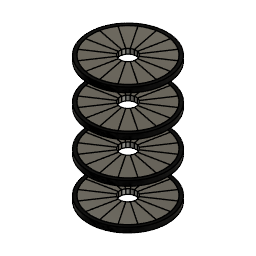
12_seal_stack_assy_set (Autodesk Fusion 360 design; units mm, degrees)
part number: 2026-05-30-09-04-55-823
Autodesk Fusion 360 part; units mm, degrees
ref_plane "WorkPlane1" through (0, 0, 50.165) normal (0, 0, 1) x (1, 0, 0)
sketch "Sketch1" plane through (0, 0, 50.165) normal (0, 0, 1) x (1, 0, 0)
  arc A0 (22.2962, -4.435) -> (22.2962, 4.435) centre (0, 0) ccw
  line L0 (22.2962, 4.435) -> (99.9218, 19.8757)
  arc A1 (99.9218, -19.8757) -> (99.9218, 19.8757) centre (0, 0) ccw
  line L1 (99.9218, -19.8757) -> (22.2962, -4.435)
extrude "Extrude1" add sketch "Sketch1" along normal blind 13.97 makes body 1
ref_plane "WorkPlane2" through (0, 0, 50.165) normal (0, 0, 1) x (1, 0, 0)
sketch "Sketch2" plane through (0, 0, 50.165) normal (0, 0, 1) x (1, 0, 0)
  arc A0 (22.2962, 4.435) -> (18.9018, 12.6298) centre (0, 0) ccw
  line L0 (18.9018, 12.6298) -> (84.7096, 56.6012)
  arc A1 (99.9218, 19.8757) -> (84.7096, 56.6012) centre (0, 0) ccw
  line L1 (99.9218, 19.8757) -> (22.2962, 4.435)
extrude "Extrude2" add sketch "Sketch2" along normal blind 13.97 separate body makes body 2
ref_plane "WorkPlane3" through (0, 0, 50.165) normal (0, 0, 1) x (1, 0, 0)
sketch "Sketch3" plane through (0, 0, 50.165) normal (0, 0, 1) x (1, 0, 0)
  arc A0 (18.9018, 12.6298) -> (12.6298, 18.9018) centre (0, 0) ccw
  line L0 (12.6298, 18.9018) -> (56.6012, 84.7096)
  arc A1 (84.7096, 56.6012) -> (56.6012, 84.7096) centre (0, 0) ccw
  line L1 (84.7096, 56.6012) -> (18.9018, 12.6298)
extrude "Extrude3" add sketch "Sketch3" along normal blind 13.97 separate body makes body 3
ref_plane "WorkPlane4" through (0, 0, 50.165) normal (0, 0, 1) x (1, 0, 0)
sketch "Sketch4" plane through (0, 0, 50.165) normal (0, 0, 1) x (1, 0, 0)
  arc A0 (12.6298, 18.9018) -> (4.435, 22.2962) centre (0, 0) ccw
  line L0 (4.435, 22.2962) -> (19.8757, 99.9218)
  arc A1 (56.6012, 84.7096) -> (19.8757, 99.9218) centre (0, 0) ccw
  line L1 (56.6012, 84.7096) -> (12.6298, 18.9018)
extrude "Extrude4" add sketch "Sketch4" along normal blind 13.97 separate body makes body 4
ref_plane "WorkPlane5" through (0, 0, 50.165) normal (0, 0, 1) x (1, 0, 0)
sketch "Sketch5" plane through (0, 0, 50.165) normal (0, 0, 1) x (1, 0, 0)
  arc A0 (4.435, 22.2962) -> (-4.435, 22.2962) centre (0, 0) ccw
  line L0 (-4.435, 22.2962) -> (-19.8757, 99.9218)
  arc A1 (19.8757, 99.9218) -> (-19.8757, 99.9218) centre (0, 0) ccw
  line L1 (19.8757, 99.9218) -> (4.435, 22.2962)
extrude "Extrude5" add sketch "Sketch5" along normal blind 13.97 separate body makes body 5
ref_plane "WorkPlane6" through (0, 0, 50.165) normal (0, 0, 1) x (1, 0, 0)
sketch "Sketch6" plane through (0, 0, 50.165) normal (0, 0, 1) x (1, 0, 0)
  arc A0 (-4.435, 22.2962) -> (-12.6298, 18.9018) centre (0, 0) ccw
  line L0 (-12.6298, 18.9018) -> (-56.6012, 84.7096)
  arc A1 (-19.8757, 99.9218) -> (-56.6012, 84.7096) centre (0, 0) ccw
  line L1 (-19.8757, 99.9218) -> (-4.435, 22.2962)
extrude "Extrude6" add sketch "Sketch6" along normal blind 13.97 separate body makes body 6
ref_plane "WorkPlane7" through (0, 0, 50.165) normal (0, 0, 1) x (1, 0, 0)
sketch "Sketch7" plane through (0, 0, 50.165) normal (0, 0, 1) x (1, 0, 0)
  arc A0 (-12.6298, 18.9018) -> (-18.9018, 12.6298) centre (0, 0) ccw
  line L0 (-18.9018, 12.6298) -> (-84.7096, 56.6012)
  arc A1 (-56.6012, 84.7096) -> (-84.7096, 56.6012) centre (0, 0) ccw
  line L1 (-56.6012, 84.7096) -> (-12.6298, 18.9018)
extrude "Extrude7" add sketch "Sketch7" along normal blind 13.97 separate body makes body 7
ref_plane "WorkPlane8" through (0, 0, 50.165) normal (0, 0, 1) x (1, 0, 0)
sketch "Sketch8" plane through (0, 0, 50.165) normal (0, 0, 1) x (1, 0, 0)
  arc A0 (-18.9018, 12.6298) -> (-22.2962, 4.435) centre (0, 0) ccw
  line L0 (-22.2962, 4.435) -> (-99.9218, 19.8757)
  arc A1 (-84.7096, 56.6012) -> (-99.9218, 19.8757) centre (0, 0) ccw
  line L1 (-84.7096, 56.6012) -> (-18.9018, 12.6298)
extrude "Extrude8" add sketch "Sketch8" along normal blind 13.97 separate body makes body 8
ref_plane "WorkPlane9" through (0, 0, 50.165) normal (0, 0, 1) x (1, 0, 0)
sketch "Sketch9" plane through (0, 0, 50.165) normal (0, 0, 1) x (1, 0, 0)
  arc A0 (-22.2962, 4.435) -> (-22.2962, -4.435) centre (0, 0) ccw
  line L0 (-22.2962, -4.435) -> (-99.9218, -19.8757)
  arc A1 (-99.9218, 19.8757) -> (-99.9218, -19.8757) centre (0, 0) ccw
  line L1 (-99.9218, 19.8757) -> (-22.2962, 4.435)
extrude "Extrude9" add sketch "Sketch9" along normal blind 13.97 separate body makes body 9
ref_plane "WorkPlane10" through (0, 0, 50.165) normal (0, 0, 1) x (1, 0, 0)
sketch "Sketch10" plane through (0, 0, 50.165) normal (0, 0, 1) x (1, 0, 0)
  arc A0 (-22.2962, -4.435) -> (-18.9018, -12.6298) centre (0, 0) ccw
  line L0 (-18.9018, -12.6298) -> (-84.7096, -56.6012)
  arc A1 (-99.9218, -19.8757) -> (-84.7096, -56.6012) centre (0, 0) ccw
  line L1 (-99.9218, -19.8757) -> (-22.2962, -4.435)
extrude "Extrude10" add sketch "Sketch10" along normal blind 13.97 separate body makes body 10
ref_plane "WorkPlane11" through (0, 0, 50.165) normal (0, 0, 1) x (1, 0, 0)
sketch "Sketch11" plane through (0, 0, 50.165) normal (0, 0, 1) x (1, 0, 0)
  arc A0 (-18.9018, -12.6298) -> (-12.6298, -18.9018) centre (0, 0) ccw
  line L0 (-12.6298, -18.9018) -> (-56.6012, -84.7096)
  arc A1 (-84.7096, -56.6012) -> (-56.6012, -84.7096) centre (0, 0) ccw
  line L1 (-84.7096, -56.6012) -> (-18.9018, -12.6298)
extrude "Extrude11" add sketch "Sketch11" along normal blind 13.97 separate body makes body 11
ref_plane "WorkPlane12" through (0, 0, 50.165) normal (0, 0, 1) x (1, 0, 0)
sketch "Sketch12" plane through (0, 0, 50.165) normal (0, 0, 1) x (1, 0, 0)
  arc A0 (-12.6298, -18.9018) -> (-4.435, -22.2962) centre (0, 0) ccw
  line L0 (-4.435, -22.2962) -> (-19.8757, -99.9218)
  arc A1 (-56.6012, -84.7096) -> (-19.8757, -99.9218) centre (0, 0) ccw
  line L1 (-56.6012, -84.7096) -> (-12.6298, -18.9018)
extrude "Extrude12" add sketch "Sketch12" along normal blind 13.97 separate body makes body 12
ref_plane "WorkPlane13" through (0, 0, 50.165) normal (0, 0, 1) x (1, 0, 0)
sketch "Sketch13" plane through (0, 0, 50.165) normal (0, 0, 1) x (1, 0, 0)
  arc A0 (-4.435, -22.2962) -> (4.435, -22.2962) centre (0, 0) ccw
  line L0 (4.435, -22.2962) -> (19.8757, -99.9218)
  arc A1 (-19.8757, -99.9218) -> (19.8757, -99.9218) centre (0, 0) ccw
  line L1 (-19.8757, -99.9218) -> (-4.435, -22.2962)
extrude "Extrude13" add sketch "Sketch13" along normal blind 13.97 separate body makes body 13
ref_plane "WorkPlane14" through (0, 0, 50.165) normal (0, 0, 1) x (1, 0, 0)
sketch "Sketch14" plane through (0, 0, 50.165) normal (0, 0, 1) x (1, 0, 0)
  arc A0 (4.435, -22.2962) -> (12.6298, -18.9018) centre (0, 0) ccw
  line L0 (12.6298, -18.9018) -> (56.6012, -84.7096)
  arc A1 (19.8757, -99.9218) -> (56.6012, -84.7096) centre (0, 0) ccw
  line L1 (19.8757, -99.9218) -> (4.435, -22.2962)
extrude "Extrude14" add sketch "Sketch14" along normal blind 13.97 separate body makes body 14
ref_plane "WorkPlane15" through (0, 0, 50.165) normal (0, 0, 1) x (1, 0, 0)
sketch "Sketch15" plane through (0, 0, 50.165) normal (0, 0, 1) x (1, 0, 0)
  arc A0 (12.6298, -18.9018) -> (18.9018, -12.6298) centre (0, 0) ccw
  line L0 (18.9018, -12.6298) -> (84.7096, -56.6012)
  arc A1 (56.6012, -84.7096) -> (84.7096, -56.6012) centre (0, 0) ccw
  line L1 (56.6012, -84.7096) -> (12.6298, -18.9018)
extrude "Extrude15" add sketch "Sketch15" along normal blind 13.97 separate body makes body 15
ref_plane "WorkPlane16" through (0, 0, 50.165) normal (0, 0, 1) x (1, 0, 0)
sketch "Sketch16" plane through (0, 0, 50.165) normal (0, 0, 1) x (1, 0, 0)
  arc A0 (18.9018, -12.6298) -> (22.2962, -4.435) centre (0, 0) ccw
  line L0 (22.2962, -4.435) -> (99.9218, -19.8757)
  arc A1 (84.7096, -56.6012) -> (99.9218, -19.8757) centre (0, 0) ccw
  line L1 (84.7096, -56.6012) -> (18.9018, -12.6298)
extrude "Extrude16" add sketch "Sketch16" along normal blind 13.97 separate body makes body 16
ref_plane "WorkPlane17" through (0, 0, 50.165) normal (0, 0, 1) x (1, 0, 0)
sketch "Sketch17" plane through (0, 0, 50.165) normal (0, 0, 1) x (1, 0, 0)
  circle A0 centre (0, 0) radius 110.744
  circle A1 centre (0, 0) radius 101.8794
extrude "Extrude17" add sketch "Sketch17" along normal blind 13.97 separate body makes body 17
ref_plane "WorkPlane18" through (0, 0, 164.465) normal (0, 0, 1) x (1, 0, 0)
sketch "Sketch18" plane through (0, 0, 164.465) normal (0, 0, 1) x (1, 0, 0)
  arc A0 (22.2962, -4.435) -> (22.2962, 4.435) centre (0, 0) ccw
  line L0 (22.2962, 4.435) -> (99.9218, 19.8757)
  arc A1 (99.9218, -19.8757) -> (99.9218, 19.8757) centre (0, 0) ccw
  line L1 (99.9218, -19.8757) -> (22.2962, -4.435)
extrude "Extrude18" add sketch "Sketch18" along normal blind 13.97 separate body makes body 18
ref_plane "WorkPlane19" through (0, 0, 164.465) normal (0, 0, 1) x (1, 0, 0)
sketch "Sketch19" plane through (0, 0, 164.465) normal (0, 0, 1) x (1, 0, 0)
  arc A0 (22.2962, 4.435) -> (18.9018, 12.6298) centre (0, 0) ccw
  line L0 (18.9018, 12.6298) -> (84.7096, 56.6012)
  arc A1 (99.9218, 19.8757) -> (84.7096, 56.6012) centre (0, 0) ccw
  line L1 (99.9218, 19.8757) -> (22.2962, 4.435)
extrude "Extrude19" add sketch "Sketch19" along normal blind 13.97 separate body makes body 19
ref_plane "WorkPlane20" through (0, 0, 164.465) normal (0, 0, 1) x (1, 0, 0)
sketch "Sketch20" plane through (0, 0, 164.465) normal (0, 0, 1) x (1, 0, 0)
  arc A0 (18.9018, 12.6298) -> (12.6298, 18.9018) centre (0, 0) ccw
  line L0 (12.6298, 18.9018) -> (56.6012, 84.7096)
  arc A1 (84.7096, 56.6012) -> (56.6012, 84.7096) centre (0, 0) ccw
  line L1 (84.7096, 56.6012) -> (18.9018, 12.6298)
extrude "Extrude20" add sketch "Sketch20" along normal blind 13.97 separate body makes body 20
ref_plane "WorkPlane21" through (0, 0, 164.465) normal (0, 0, 1) x (1, 0, 0)
sketch "Sketch21" plane through (0, 0, 164.465) normal (0, 0, 1) x (1, 0, 0)
  arc A0 (12.6298, 18.9018) -> (4.435, 22.2962) centre (0, 0) ccw
  line L0 (4.435, 22.2962) -> (19.8757, 99.9218)
  arc A1 (56.6012, 84.7096) -> (19.8757, 99.9218) centre (0, 0) ccw
  line L1 (56.6012, 84.7096) -> (12.6298, 18.9018)
extrude "Extrude21" add sketch "Sketch21" along normal blind 13.97 separate body makes body 21
ref_plane "WorkPlane22" through (0, 0, 164.465) normal (0, 0, 1) x (1, 0, 0)
sketch "Sketch22" plane through (0, 0, 164.465) normal (0, 0, 1) x (1, 0, 0)
  arc A0 (4.435, 22.2962) -> (-4.435, 22.2962) centre (0, 0) ccw
  line L0 (-4.435, 22.2962) -> (-19.8757, 99.9218)
  arc A1 (19.8757, 99.9218) -> (-19.8757, 99.9218) centre (0, 0) ccw
  line L1 (19.8757, 99.9218) -> (4.435, 22.2962)
extrude "Extrude22" add sketch "Sketch22" along normal blind 13.97 separate body makes body 22
ref_plane "WorkPlane23" through (0, 0, 164.465) normal (0, 0, 1) x (1, 0, 0)
sketch "Sketch23" plane through (0, 0, 164.465) normal (0, 0, 1) x (1, 0, 0)
  arc A0 (-4.435, 22.2962) -> (-12.6298, 18.9018) centre (0, 0) ccw
  line L0 (-12.6298, 18.9018) -> (-56.6012, 84.7096)
  arc A1 (-19.8757, 99.9218) -> (-56.6012, 84.7096) centre (0, 0) ccw
  line L1 (-19.8757, 99.9218) -> (-4.435, 22.2962)
extrude "Extrude23" add sketch "Sketch23" along normal blind 13.97 separate body makes body 23
ref_plane "WorkPlane24" through (0, 0, 164.465) normal (0, 0, 1) x (1, 0, 0)
sketch "Sketch24" plane through (0, 0, 164.465) normal (0, 0, 1) x (1, 0, 0)
  arc A0 (-12.6298, 18.9018) -> (-18.9018, 12.6298) centre (0, 0) ccw
  line L0 (-18.9018, 12.6298) -> (-84.7096, 56.6012)
  arc A1 (-56.6012, 84.7096) -> (-84.7096, 56.6012) centre (0, 0) ccw
  line L1 (-56.6012, 84.7096) -> (-12.6298, 18.9018)
extrude "Extrude24" add sketch "Sketch24" along normal blind 13.97 separate body makes body 24
ref_plane "WorkPlane25" through (0, 0, 164.465) normal (0, 0, 1) x (1, 0, 0)
sketch "Sketch25" plane through (0, 0, 164.465) normal (0, 0, 1) x (1, 0, 0)
  arc A0 (-18.9018, 12.6298) -> (-22.2962, 4.435) centre (0, 0) ccw
  line L0 (-22.2962, 4.435) -> (-99.9218, 19.8757)
  arc A1 (-84.7096, 56.6012) -> (-99.9218, 19.8757) centre (0, 0) ccw
  line L1 (-84.7096, 56.6012) -> (-18.9018, 12.6298)
extrude "Extrude25" add sketch "Sketch25" along normal blind 13.97 separate body makes body 25
ref_plane "WorkPlane26" through (0, 0, 164.465) normal (0, 0, 1) x (1, 0, 0)
sketch "Sketch26" plane through (0, 0, 164.465) normal (0, 0, 1) x (1, 0, 0)
  arc A0 (-22.2962, 4.435) -> (-22.2962, -4.435) centre (0, 0) ccw
  line L0 (-22.2962, -4.435) -> (-99.9218, -19.8757)
  arc A1 (-99.9218, 19.8757) -> (-99.9218, -19.8757) centre (0, 0) ccw
  line L1 (-99.9218, 19.8757) -> (-22.2962, 4.435)
extrude "Extrude26" add sketch "Sketch26" along normal blind 13.97 separate body makes body 26
ref_plane "WorkPlane27" through (0, 0, 164.465) normal (0, 0, 1) x (1, 0, 0)
sketch "Sketch27" plane through (0, 0, 164.465) normal (0, 0, 1) x (1, 0, 0)
  arc A0 (-22.2962, -4.435) -> (-18.9018, -12.6298) centre (0, 0) ccw
  line L0 (-18.9018, -12.6298) -> (-84.7096, -56.6012)
  arc A1 (-99.9218, -19.8757) -> (-84.7096, -56.6012) centre (0, 0) ccw
  line L1 (-99.9218, -19.8757) -> (-22.2962, -4.435)
extrude "Extrude27" add sketch "Sketch27" along normal blind 13.97 separate body makes body 27
ref_plane "WorkPlane28" through (0, 0, 164.465) normal (0, 0, 1) x (1, 0, 0)
sketch "Sketch28" plane through (0, 0, 164.465) normal (0, 0, 1) x (1, 0, 0)
  arc A0 (-18.9018, -12.6298) -> (-12.6298, -18.9018) centre (0, 0) ccw
  line L0 (-12.6298, -18.9018) -> (-56.6012, -84.7096)
  arc A1 (-84.7096, -56.6012) -> (-56.6012, -84.7096) centre (0, 0) ccw
  line L1 (-84.7096, -56.6012) -> (-18.9018, -12.6298)
extrude "Extrude28" add sketch "Sketch28" along normal blind 13.97 separate body makes body 28
ref_plane "WorkPlane29" through (0, 0, 164.465) normal (0, 0, 1) x (1, 0, 0)
sketch "Sketch29" plane through (0, 0, 164.465) normal (0, 0, 1) x (1, 0, 0)
  arc A0 (-12.6298, -18.9018) -> (-4.435, -22.2962) centre (0, 0) ccw
  line L0 (-4.435, -22.2962) -> (-19.8757, -99.9218)
  arc A1 (-56.6012, -84.7096) -> (-19.8757, -99.9218) centre (0, 0) ccw
  line L1 (-56.6012, -84.7096) -> (-12.6298, -18.9018)
extrude "Extrude29" add sketch "Sketch29" along normal blind 13.97 separate body makes body 29
ref_plane "WorkPlane30" through (0, 0, 164.465) normal (0, 0, 1) x (1, 0, 0)
sketch "Sketch30" plane through (0, 0, 164.465) normal (0, 0, 1) x (1, 0, 0)
  arc A0 (-4.435, -22.2962) -> (4.435, -22.2962) centre (0, 0) ccw
  line L0 (4.435, -22.2962) -> (19.8757, -99.9218)
  arc A1 (-19.8757, -99.9218) -> (19.8757, -99.9218) centre (0, 0) ccw
  line L1 (-19.8757, -99.9218) -> (-4.435, -22.2962)
extrude "Extrude30" add sketch "Sketch30" along normal blind 13.97 separate body makes body 30
ref_plane "WorkPlane31" through (0, 0, 164.465) normal (0, 0, 1) x (1, 0, 0)
sketch "Sketch31" plane through (0, 0, 164.465) normal (0, 0, 1) x (1, 0, 0)
  arc A0 (4.435, -22.2962) -> (12.6298, -18.9018) centre (0, 0) ccw
  line L0 (12.6298, -18.9018) -> (56.6012, -84.7096)
  arc A1 (19.8757, -99.9218) -> (56.6012, -84.7096) centre (0, 0) ccw
  line L1 (19.8757, -99.9218) -> (4.435, -22.2962)
extrude "Extrude31" add sketch "Sketch31" along normal blind 13.97 separate body makes body 31
ref_plane "WorkPlane32" through (0, 0, 164.465) normal (0, 0, 1) x (1, 0, 0)
sketch "Sketch32" plane through (0, 0, 164.465) normal (0, 0, 1) x (1, 0, 0)
  arc A0 (12.6298, -18.9018) -> (18.9018, -12.6298) centre (0, 0) ccw
  line L0 (18.9018, -12.6298) -> (84.7096, -56.6012)
  arc A1 (56.6012, -84.7096) -> (84.7096, -56.6012) centre (0, 0) ccw
  line L1 (56.6012, -84.7096) -> (12.6298, -18.9018)
extrude "Extrude32" add sketch "Sketch32" along normal blind 13.97 separate body makes body 32
ref_plane "WorkPlane33" through (0, 0, 164.465) normal (0, 0, 1) x (1, 0, 0)
sketch "Sketch33" plane through (0, 0, 164.465) normal (0, 0, 1) x (1, 0, 0)
  arc A0 (18.9018, -12.6298) -> (22.2962, -4.435) centre (0, 0) ccw
  line L0 (22.2962, -4.435) -> (99.9218, -19.8757)
  arc A1 (84.7096, -56.6012) -> (99.9218, -19.8757) centre (0, 0) ccw
  line L1 (84.7096, -56.6012) -> (18.9018, -12.6298)
extrude "Extrude33" add sketch "Sketch33" along normal blind 13.97 separate body makes body 33
ref_plane "WorkPlane34" through (0, 0, 164.465) normal (0, 0, 1) x (1, 0, 0)
sketch "Sketch34" plane through (0, 0, 164.465) normal (0, 0, 1) x (1, 0, 0)
  circle A0 centre (0, 0) radius 110.744
  circle A1 centre (0, 0) radius 101.8794
extrude "Extrude34" add sketch "Sketch34" along normal blind 13.97 separate body makes body 34
ref_plane "WorkPlane35" through (0, 0, 278.765) normal (0, 0, 1) x (1, 0, 0)
sketch "Sketch35" plane through (0, 0, 278.765) normal (0, 0, 1) x (1, 0, 0)
  arc A0 (22.2962, -4.435) -> (22.2962, 4.435) centre (0, 0) ccw
  line L0 (22.2962, 4.435) -> (99.9218, 19.8757)
  arc A1 (99.9218, -19.8757) -> (99.9218, 19.8757) centre (0, 0) ccw
  line L1 (99.9218, -19.8757) -> (22.2962, -4.435)
extrude "Extrude35" add sketch "Sketch35" along normal blind 13.97 separate body makes body 35
ref_plane "WorkPlane36" through (0, 0, 278.765) normal (0, 0, 1) x (1, 0, 0)
sketch "Sketch36" plane through (0, 0, 278.765) normal (0, 0, 1) x (1, 0, 0)
  arc A0 (22.2962, 4.435) -> (18.9018, 12.6298) centre (0, 0) ccw
  line L0 (18.9018, 12.6298) -> (84.7096, 56.6012)
  arc A1 (99.9218, 19.8757) -> (84.7096, 56.6012) centre (0, 0) ccw
  line L1 (99.9218, 19.8757) -> (22.2962, 4.435)
extrude "Extrude36" add sketch "Sketch36" along normal blind 13.97 separate body makes body 36
ref_plane "WorkPlane37" through (0, 0, 278.765) normal (0, 0, 1) x (1, 0, 0)
sketch "Sketch37" plane through (0, 0, 278.765) normal (0, 0, 1) x (1, 0, 0)
  arc A0 (18.9018, 12.6298) -> (12.6298, 18.9018) centre (0, 0) ccw
  line L0 (12.6298, 18.9018) -> (56.6012, 84.7096)
  arc A1 (84.7096, 56.6012) -> (56.6012, 84.7096) centre (0, 0) ccw
  line L1 (84.7096, 56.6012) -> (18.9018, 12.6298)
extrude "Extrude37" add sketch "Sketch37" along normal blind 13.97 separate body makes body 37
ref_plane "WorkPlane38" through (0, 0, 278.765) normal (0, 0, 1) x (1, 0, 0)
sketch "Sketch38" plane through (0, 0, 278.765) normal (0, 0, 1) x (1, 0, 0)
  arc A0 (12.6298, 18.9018) -> (4.435, 22.2962) centre (0, 0) ccw
  line L0 (4.435, 22.2962) -> (19.8757, 99.9218)
  arc A1 (56.6012, 84.7096) -> (19.8757, 99.9218) centre (0, 0) ccw
  line L1 (56.6012, 84.7096) -> (12.6298, 18.9018)
extrude "Extrude38" add sketch "Sketch38" along normal blind 13.97 separate body makes body 38
ref_plane "WorkPlane39" through (0, 0, 278.765) normal (0, 0, 1) x (1, 0, 0)
sketch "Sketch39" plane through (0, 0, 278.765) normal (0, 0, 1) x (1, 0, 0)
  arc A0 (4.435, 22.2962) -> (-4.435, 22.2962) centre (0, 0) ccw
  line L0 (-4.435, 22.2962) -> (-19.8757, 99.9218)
  arc A1 (19.8757, 99.9218) -> (-19.8757, 99.9218) centre (0, 0) ccw
  line L1 (19.8757, 99.9218) -> (4.435, 22.2962)
extrude "Extrude39" add sketch "Sketch39" along normal blind 13.97 separate body makes body 39
ref_plane "WorkPlane40" through (0, 0, 278.765) normal (0, 0, 1) x (1, 0, 0)
sketch "Sketch40" plane through (0, 0, 278.765) normal (0, 0, 1) x (1, 0, 0)
  arc A0 (-4.435, 22.2962) -> (-12.6298, 18.9018) centre (0, 0) ccw
  line L0 (-12.6298, 18.9018) -> (-56.6012, 84.7096)
  arc A1 (-19.8757, 99.9218) -> (-56.6012, 84.7096) centre (0, 0) ccw
  line L1 (-19.8757, 99.9218) -> (-4.435, 22.2962)
extrude "Extrude40" add sketch "Sketch40" along normal blind 13.97 separate body makes body 40
ref_plane "WorkPlane41" through (0, 0, 278.765) normal (0, 0, 1) x (1, 0, 0)
sketch "Sketch41" plane through (0, 0, 278.765) normal (0, 0, 1) x (1, 0, 0)
  arc A0 (-12.6298, 18.9018) -> (-18.9018, 12.6298) centre (0, 0) ccw
  line L0 (-18.9018, 12.6298) -> (-84.7096, 56.6012)
  arc A1 (-56.6012, 84.7096) -> (-84.7096, 56.6012) centre (0, 0) ccw
  line L1 (-56.6012, 84.7096) -> (-12.6298, 18.9018)
extrude "Extrude41" add sketch "Sketch41" along normal blind 13.97 separate body makes body 41
ref_plane "WorkPlane42" through (0, 0, 278.765) normal (0, 0, 1) x (1, 0, 0)
sketch "Sketch42" plane through (0, 0, 278.765) normal (0, 0, 1) x (1, 0, 0)
  arc A0 (-18.9018, 12.6298) -> (-22.2962, 4.435) centre (0, 0) ccw
  line L0 (-22.2962, 4.435) -> (-99.9218, 19.8757)
  arc A1 (-84.7096, 56.6012) -> (-99.9218, 19.8757) centre (0, 0) ccw
  line L1 (-84.7096, 56.6012) -> (-18.9018, 12.6298)
extrude "Extrude42" add sketch "Sketch42" along normal blind 13.97 separate body makes body 42
ref_plane "WorkPlane43" through (0, 0, 278.765) normal (0, 0, 1) x (1, 0, 0)
sketch "Sketch43" plane through (0, 0, 278.765) normal (0, 0, 1) x (1, 0, 0)
  arc A0 (-22.2962, 4.435) -> (-22.2962, -4.435) centre (0, 0) ccw
  line L0 (-22.2962, -4.435) -> (-99.9218, -19.8757)
  arc A1 (-99.9218, 19.8757) -> (-99.9218, -19.8757) centre (0, 0) ccw
  line L1 (-99.9218, 19.8757) -> (-22.2962, 4.435)
extrude "Extrude43" add sketch "Sketch43" along normal blind 13.97 separate body makes body 43
ref_plane "WorkPlane44" through (0, 0, 278.765) normal (0, 0, 1) x (1, 0, 0)
sketch "Sketch44" plane through (0, 0, 278.765) normal (0, 0, 1) x (1, 0, 0)
  arc A0 (-22.2962, -4.435) -> (-18.9018, -12.6298) centre (0, 0) ccw
  line L0 (-18.9018, -12.6298) -> (-84.7096, -56.6012)
  arc A1 (-99.9218, -19.8757) -> (-84.7096, -56.6012) centre (0, 0) ccw
  line L1 (-99.9218, -19.8757) -> (-22.2962, -4.435)
extrude "Extrude44" add sketch "Sketch44" along normal blind 13.97 separate body makes body 44
ref_plane "WorkPlane45" through (0, 0, 278.765) normal (0, 0, 1) x (1, 0, 0)
sketch "Sketch45" plane through (0, 0, 278.765) normal (0, 0, 1) x (1, 0, 0)
  arc A0 (-18.9018, -12.6298) -> (-12.6298, -18.9018) centre (0, 0) ccw
  line L0 (-12.6298, -18.9018) -> (-56.6012, -84.7096)
  arc A1 (-84.7096, -56.6012) -> (-56.6012, -84.7096) centre (0, 0) ccw
  line L1 (-84.7096, -56.6012) -> (-18.9018, -12.6298)
extrude "Extrude45" add sketch "Sketch45" along normal blind 13.97 separate body makes body 45
ref_plane "WorkPlane46" through (0, 0, 278.765) normal (0, 0, 1) x (1, 0, 0)
sketch "Sketch46" plane through (0, 0, 278.765) normal (0, 0, 1) x (1, 0, 0)
  arc A0 (-12.6298, -18.9018) -> (-4.435, -22.2962) centre (0, 0) ccw
  line L0 (-4.435, -22.2962) -> (-19.8757, -99.9218)
  arc A1 (-56.6012, -84.7096) -> (-19.8757, -99.9218) centre (0, 0) ccw
  line L1 (-56.6012, -84.7096) -> (-12.6298, -18.9018)
extrude "Extrude46" add sketch "Sketch46" along normal blind 13.97 separate body makes body 46
ref_plane "WorkPlane47" through (0, 0, 278.765) normal (0, 0, 1) x (1, 0, 0)
sketch "Sketch47" plane through (0, 0, 278.765) normal (0, 0, 1) x (1, 0, 0)
  arc A0 (-4.435, -22.2962) -> (4.435, -22.2962) centre (0, 0) ccw
  line L0 (4.435, -22.2962) -> (19.8757, -99.9218)
  arc A1 (-19.8757, -99.9218) -> (19.8757, -99.9218) centre (0, 0) ccw
  line L1 (-19.8757, -99.9218) -> (-4.435, -22.2962)
extrude "Extrude47" add sketch "Sketch47" along normal blind 13.97 separate body makes body 47
ref_plane "WorkPlane48" through (0, 0, 278.765) normal (0, 0, 1) x (1, 0, 0)
sketch "Sketch48" plane through (0, 0, 278.765) normal (0, 0, 1) x (1, 0, 0)
  arc A0 (4.435, -22.2962) -> (12.6298, -18.9018) centre (0, 0) ccw
  line L0 (12.6298, -18.9018) -> (56.6012, -84.7096)
  arc A1 (19.8757, -99.9218) -> (56.6012, -84.7096) centre (0, 0) ccw
  line L1 (19.8757, -99.9218) -> (4.435, -22.2962)
extrude "Extrude48" add sketch "Sketch48" along normal blind 13.97 separate body makes body 48
ref_plane "WorkPlane49" through (0, 0, 278.765) normal (0, 0, 1) x (1, 0, 0)
sketch "Sketch49" plane through (0, 0, 278.765) normal (0, 0, 1) x (1, 0, 0)
  arc A0 (12.6298, -18.9018) -> (18.9018, -12.6298) centre (0, 0) ccw
  line L0 (18.9018, -12.6298) -> (84.7096, -56.6012)
  arc A1 (56.6012, -84.7096) -> (84.7096, -56.6012) centre (0, 0) ccw
  line L1 (56.6012, -84.7096) -> (12.6298, -18.9018)
extrude "Extrude49" add sketch "Sketch49" along normal blind 13.97 separate body makes body 49
ref_plane "WorkPlane50" through (0, 0, 278.765) normal (0, 0, 1) x (1, 0, 0)
sketch "Sketch50" plane through (0, 0, 278.765) normal (0, 0, 1) x (1, 0, 0)
  arc A0 (18.9018, -12.6298) -> (22.2962, -4.435) centre (0, 0) ccw
  line L0 (22.2962, -4.435) -> (99.9218, -19.8757)
  arc A1 (84.7096, -56.6012) -> (99.9218, -19.8757) centre (0, 0) ccw
  line L1 (84.7096, -56.6012) -> (18.9018, -12.6298)
extrude "Extrude50" add sketch "Sketch50" along normal blind 13.97 separate body makes body 50
ref_plane "WorkPlane51" through (0, 0, 278.765) normal (0, 0, 1) x (1, 0, 0)
sketch "Sketch51" plane through (0, 0, 278.765) normal (0, 0, 1) x (1, 0, 0)
  circle A0 centre (0, 0) radius 110.744
  circle A1 centre (0, 0) radius 101.8794
extrude "Extrude51" add sketch "Sketch51" along normal blind 13.97 separate body makes body 51
ref_plane "WorkPlane52" through (0, 0, 393.065) normal (0, 0, 1) x (1, 0, 0)
sketch "Sketch52" plane through (0, 0, 393.065) normal (0, 0, 1) x (1, 0, 0)
  arc A0 (22.2962, -4.435) -> (22.2962, 4.435) centre (0, 0) ccw
  line L0 (22.2962, 4.435) -> (99.9218, 19.8757)
  arc A1 (99.9218, -19.8757) -> (99.9218, 19.8757) centre (0, 0) ccw
  line L1 (99.9218, -19.8757) -> (22.2962, -4.435)
extrude "Extrude52" add sketch "Sketch52" along normal blind 13.97 separate body makes body 52
ref_plane "WorkPlane53" through (0, 0, 393.065) normal (0, 0, 1) x (1, 0, 0)
sketch "Sketch53" plane through (0, 0, 393.065) normal (0, 0, 1) x (1, 0, 0)
  arc A0 (22.2962, 4.435) -> (18.9018, 12.6298) centre (0, 0) ccw
  line L0 (18.9018, 12.6298) -> (84.7096, 56.6012)
  arc A1 (99.9218, 19.8757) -> (84.7096, 56.6012) centre (0, 0) ccw
  line L1 (99.9218, 19.8757) -> (22.2962, 4.435)
extrude "Extrude53" add sketch "Sketch53" along normal blind 13.97 separate body makes body 53
ref_plane "WorkPlane54" through (0, 0, 393.065) normal (0, 0, 1) x (1, 0, 0)
sketch "Sketch54" plane through (0, 0, 393.065) normal (0, 0, 1) x (1, 0, 0)
  arc A0 (18.9018, 12.6298) -> (12.6298, 18.9018) centre (0, 0) ccw
  line L0 (12.6298, 18.9018) -> (56.6012, 84.7096)
  arc A1 (84.7096, 56.6012) -> (56.6012, 84.7096) centre (0, 0) ccw
  line L1 (84.7096, 56.6012) -> (18.9018, 12.6298)
extrude "Extrude54" add sketch "Sketch54" along normal blind 13.97 separate body makes body 54
ref_plane "WorkPlane55" through (0, 0, 393.065) normal (0, 0, 1) x (1, 0, 0)
sketch "Sketch55" plane through (0, 0, 393.065) normal (0, 0, 1) x (1, 0, 0)
  arc A0 (12.6298, 18.9018) -> (4.435, 22.2962) centre (0, 0) ccw
  line L0 (4.435, 22.2962) -> (19.8757, 99.9218)
  arc A1 (56.6012, 84.7096) -> (19.8757, 99.9218) centre (0, 0) ccw
  line L1 (56.6012, 84.7096) -> (12.6298, 18.9018)
extrude "Extrude55" add sketch "Sketch55" along normal blind 13.97 separate body makes body 55
ref_plane "WorkPlane56" through (0, 0, 393.065) normal (0, 0, 1) x (1, 0, 0)
sketch "Sketch56" plane through (0, 0, 393.065) normal (0, 0, 1) x (1, 0, 0)
  arc A0 (4.435, 22.2962) -> (-4.435, 22.2962) centre (0, 0) ccw
  line L0 (-4.435, 22.2962) -> (-19.8757, 99.9218)
  arc A1 (19.8757, 99.9218) -> (-19.8757, 99.9218) centre (0, 0) ccw
  line L1 (19.8757, 99.9218) -> (4.435, 22.2962)
extrude "Extrude56" add sketch "Sketch56" along normal blind 13.97 separate body makes body 56
ref_plane "WorkPlane57" through (0, 0, 393.065) normal (0, 0, 1) x (1, 0, 0)
sketch "Sketch57" plane through (0, 0, 393.065) normal (0, 0, 1) x (1, 0, 0)
  arc A0 (-4.435, 22.2962) -> (-12.6298, 18.9018) centre (0, 0) ccw
  line L0 (-12.6298, 18.9018) -> (-56.6012, 84.7096)
  arc A1 (-19.8757, 99.9218) -> (-56.6012, 84.7096) centre (0, 0) ccw
  line L1 (-19.8757, 99.9218) -> (-4.435, 22.2962)
extrude "Extrude57" add sketch "Sketch57" along normal blind 13.97 separate body makes body 57
ref_plane "WorkPlane58" through (0, 0, 393.065) normal (0, 0, 1) x (1, 0, 0)
sketch "Sketch58" plane through (0, 0, 393.065) normal (0, 0, 1) x (1, 0, 0)
  arc A0 (-12.6298, 18.9018) -> (-18.9018, 12.6298) centre (0, 0) ccw
  line L0 (-18.9018, 12.6298) -> (-84.7096, 56.6012)
  arc A1 (-56.6012, 84.7096) -> (-84.7096, 56.6012) centre (0, 0) ccw
  line L1 (-56.6012, 84.7096) -> (-12.6298, 18.9018)
extrude "Extrude58" add sketch "Sketch58" along normal blind 13.97 separate body makes body 58
ref_plane "WorkPlane59" through (0, 0, 393.065) normal (0, 0, 1) x (1, 0, 0)
sketch "Sketch59" plane through (0, 0, 393.065) normal (0, 0, 1) x (1, 0, 0)
  arc A0 (-18.9018, 12.6298) -> (-22.2962, 4.435) centre (0, 0) ccw
  line L0 (-22.2962, 4.435) -> (-99.9218, 19.8757)
  arc A1 (-84.7096, 56.6012) -> (-99.9218, 19.8757) centre (0, 0) ccw
  line L1 (-84.7096, 56.6012) -> (-18.9018, 12.6298)
extrude "Extrude59" add sketch "Sketch59" along normal blind 13.97 separate body makes body 59
ref_plane "WorkPlane60" through (0, 0, 393.065) normal (0, 0, 1) x (1, 0, 0)
sketch "Sketch60" plane through (0, 0, 393.065) normal (0, 0, 1) x (1, 0, 0)
  arc A0 (-22.2962, 4.435) -> (-22.2962, -4.435) centre (0, 0) ccw
  line L0 (-22.2962, -4.435) -> (-99.9218, -19.8757)
  arc A1 (-99.9218, 19.8757) -> (-99.9218, -19.8757) centre (0, 0) ccw
  line L1 (-99.9218, 19.8757) -> (-22.2962, 4.435)
extrude "Extrude60" add sketch "Sketch60" along normal blind 13.97 separate body makes body 60
ref_plane "WorkPlane61" through (0, 0, 393.065) normal (0, 0, 1) x (1, 0, 0)
sketch "Sketch61" plane through (0, 0, 393.065) normal (0, 0, 1) x (1, 0, 0)
  arc A0 (-22.2962, -4.435) -> (-18.9018, -12.6298) centre (0, 0) ccw
  line L0 (-18.9018, -12.6298) -> (-84.7096, -56.6012)
  arc A1 (-99.9218, -19.8757) -> (-84.7096, -56.6012) centre (0, 0) ccw
  line L1 (-99.9218, -19.8757) -> (-22.2962, -4.435)
extrude "Extrude61" add sketch "Sketch61" along normal blind 13.97 separate body makes body 61
ref_plane "WorkPlane62" through (0, 0, 393.065) normal (0, 0, 1) x (1, 0, 0)
sketch "Sketch62" plane through (0, 0, 393.065) normal (0, 0, 1) x (1, 0, 0)
  arc A0 (-18.9018, -12.6298) -> (-12.6298, -18.9018) centre (0, 0) ccw
  line L0 (-12.6298, -18.9018) -> (-56.6012, -84.7096)
  arc A1 (-84.7096, -56.6012) -> (-56.6012, -84.7096) centre (0, 0) ccw
  line L1 (-84.7096, -56.6012) -> (-18.9018, -12.6298)
extrude "Extrude62" add sketch "Sketch62" along normal blind 13.97 separate body makes body 62
ref_plane "WorkPlane63" through (0, 0, 393.065) normal (0, 0, 1) x (1, 0, 0)
sketch "Sketch63" plane through (0, 0, 393.065) normal (0, 0, 1) x (1, 0, 0)
  arc A0 (-12.6298, -18.9018) -> (-4.435, -22.2962) centre (0, 0) ccw
  line L0 (-4.435, -22.2962) -> (-19.8757, -99.9218)
  arc A1 (-56.6012, -84.7096) -> (-19.8757, -99.9218) centre (0, 0) ccw
  line L1 (-56.6012, -84.7096) -> (-12.6298, -18.9018)
extrude "Extrude63" add sketch "Sketch63" along normal blind 13.97 separate body makes body 63
ref_plane "WorkPlane64" through (0, 0, 393.065) normal (0, 0, 1) x (1, 0, 0)
sketch "Sketch64" plane through (0, 0, 393.065) normal (0, 0, 1) x (1, 0, 0)
  arc A0 (-4.435, -22.2962) -> (4.435, -22.2962) centre (0, 0) ccw
  line L0 (4.435, -22.2962) -> (19.8757, -99.9218)
  arc A1 (-19.8757, -99.9218) -> (19.8757, -99.9218) centre (0, 0) ccw
  line L1 (-19.8757, -99.9218) -> (-4.435, -22.2962)
extrude "Extrude64" add sketch "Sketch64" along normal blind 13.97 separate body makes body 64
ref_plane "WorkPlane65" through (0, 0, 393.065) normal (0, 0, 1) x (1, 0, 0)
sketch "Sketch65" plane through (0, 0, 393.065) normal (0, 0, 1) x (1, 0, 0)
  arc A0 (4.435, -22.2962) -> (12.6298, -18.9018) centre (0, 0) ccw
  line L0 (12.6298, -18.9018) -> (56.6012, -84.7096)
  arc A1 (19.8757, -99.9218) -> (56.6012, -84.7096) centre (0, 0) ccw
  line L1 (19.8757, -99.9218) -> (4.435, -22.2962)
extrude "Extrude65" add sketch "Sketch65" along normal blind 13.97 separate body makes body 65
ref_plane "WorkPlane66" through (0, 0, 393.065) normal (0, 0, 1) x (1, 0, 0)
sketch "Sketch66" plane through (0, 0, 393.065) normal (0, 0, 1) x (1, 0, 0)
  arc A0 (12.6298, -18.9018) -> (18.9018, -12.6298) centre (0, 0) ccw
  line L0 (18.9018, -12.6298) -> (84.7096, -56.6012)
  arc A1 (56.6012, -84.7096) -> (84.7096, -56.6012) centre (0, 0) ccw
  line L1 (56.6012, -84.7096) -> (12.6298, -18.9018)
extrude "Extrude66" add sketch "Sketch66" along normal blind 13.97 separate body makes body 66
ref_plane "WorkPlane67" through (0, 0, 393.065) normal (0, 0, 1) x (1, 0, 0)
sketch "Sketch67" plane through (0, 0, 393.065) normal (0, 0, 1) x (1, 0, 0)
  arc A0 (18.9018, -12.6298) -> (22.2962, -4.435) centre (0, 0) ccw
  line L0 (22.2962, -4.435) -> (99.9218, -19.8757)
  arc A1 (84.7096, -56.6012) -> (99.9218, -19.8757) centre (0, 0) ccw
  line L1 (84.7096, -56.6012) -> (18.9018, -12.6298)
extrude "Extrude67" add sketch "Sketch67" along normal blind 13.97 separate body makes body 67
ref_plane "WorkPlane68" through (0, 0, 393.065) normal (0, 0, 1) x (1, 0, 0)
sketch "Sketch68" plane through (0, 0, 393.065) normal (0, 0, 1) x (1, 0, 0)
  circle A0 centre (0, 0) radius 110.744
  circle A1 centre (0, 0) radius 101.8794
extrude "Extrude68" add sketch "Sketch68" along normal blind 13.97 separate body makes body 68
named bodies: "SHEX-005_petal_L1_01", "SHEX-005_petal_L1_02", "SHEX-005_petal_L1_03", "SHEX-005_petal_L1_04", "SHEX-005_petal_L1_05", "SHEX-005_petal_L1_06", "SHEX-005_petal_L1_07", "SHEX-005_petal_L1_08", "SHEX-005_petal_L1_09", "SHEX-005_petal_L1_10", "SHEX-005_petal_L1_11", "SHEX-005_petal_L1_12", "SHEX-005_petal_L1_13", "SHEX-005_petal_L1_14", "SHEX-005_petal_L1_15", "SHEX-005_petal_L1_16", "SHEX-004_cup_L1", "SHEX-005_petal_L2_01", "SHEX-005_petal_L2_02", "SHEX-005_petal_L2_03", "SHEX-005_petal_L2_04", "SHEX-005_petal_L2_05", "SHEX-005_petal_L2_06", "SHEX-005_petal_L2_07", "SHEX-005_petal_L2_08", "SHEX-005_petal_L2_09", "SHEX-005_petal_L2_10", "SHEX-005_petal_L2_11", "SHEX-005_petal_L2_12", "SHEX-005_petal_L2_13", "SHEX-005_petal_L2_14", "SHEX-005_petal_L2_15", "SHEX-005_petal_L2_16", "SHEX-004_cup_L2", "SHEX-005_petal_L3_01", "SHEX-005_petal_L3_02", "SHEX-005_petal_L3_03", "SHEX-005_petal_L3_04", "SHEX-005_petal_L3_05", "SHEX-005_petal_L3_06", "SHEX-005_petal_L3_07", "SHEX-005_petal_L3_08", "SHEX-005_petal_L3_09", "SHEX-005_petal_L3_10", "SHEX-005_petal_L3_11", "SHEX-005_petal_L3_12", "SHEX-005_petal_L3_13", "SHEX-005_petal_L3_14", "SHEX-005_petal_L3_15", "SHEX-005_petal_L3_16", "SHEX-004_cup_L3", "SHEX-005_petal_L4_01", "SHEX-005_petal_L4_02", "SHEX-005_petal_L4_03", "SHEX-005_petal_L4_04", "SHEX-005_petal_L4_05", "SHEX-005_petal_L4_06", "SHEX-005_petal_L4_07", "SHEX-005_petal_L4_08", "SHEX-005_petal_L4_09", "SHEX-005_petal_L4_10", "SHEX-005_petal_L4_11", "SHEX-005_petal_L4_12", "SHEX-005_petal_L4_13", "SHEX-005_petal_L4_14", "SHEX-005_petal_L4_15", "SHEX-005_petal_L4_16", "SHEX-004_cup_L4"
